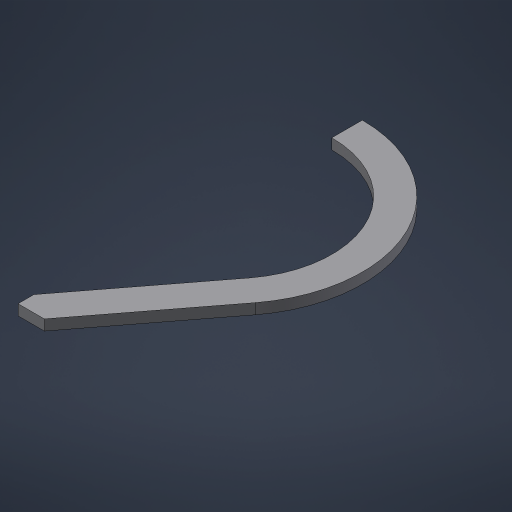
# Autodesk Inventor part: LEDholderv
Saved by Autodesk Inventor 2023.5 (Build 275446000, 446)
## iProperties
Created: 2025-03-20
Part Number: LEDholderv
Material: Generisch
Document SubType Name: Modeling
Designer: David Lill
Density: 1 g/cm^3
Appearance: Vorgabe
Author: David Lill
## iProperties of the stored document LEDholderv_3D-Druck.ipt
Part Number: LEDholderv_3D-Druck
Material: Allgemein
Document SubType Name: Modellieren
Designer: David Lill
Appearance: Vorgabe
Author: David Lill
Autodesk Inventor part; units mm, degrees
ref_plane "YZ Plane" through (0, 0, 0) normal (1, 0, 0) x (0, 1, 0)
ref_plane "XZ Plane" through (0, 0, 0) normal (0, 1, 0) x (-1, 0, 0)
ref_plane "XY Plane" through (0, 0, 0) normal (0, 0, 1) x (1, 0, 0)
sketch "Skizze1" plane through (0, 0, 0) normal (0, 0, 1) x (1, 0, 0)
  line L0 (0, 0) -> (5, 0)
  line L1 (5, 0) -> (22.3624, 22.7154)
  arc A0 (22.3624, 22.7154) -> (2.5, 62.8971) centre (2.5, 37.8971) ccw
  line L2 (2.5, 62.8971) -> (2.5, 57.1029)
  arc A1 (17.7589, 26.2341) -> (2.5, 57.1029) centre (2.5, 37.8971) ccw
  line L3 (17.7589, 26.2341) -> (0, 3)
  line L4 (0, 3) -> (0, 0)
  point P0 (2.5, 0)
  point P1 (2.5, 60)
  dimension "d0" = 3
  dimension "d1" = 5
  dimension "d2" = 25
  dimension "d3" = 60
  constraints: 10 end point, 4 point on circle, 2 centre point, 2 midpoint, 2 parallel, 2 tangent, 1 concentric, 1 horizontal, 1 perpendicular, 1 point on line, 1 vertical alignment
  measures "d0" distance of L3.end L0.start
  measures "d1" distance of L0.start L0.end
  measures "d2" radius of A0
  measures "d3" distance from line of L0 point (2.5, 60)
extrude "Extrusion1" add sketch "Skizze1" along normal blind 2
